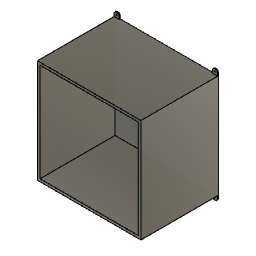
caixinha morea v0 (Autodesk Fusion 360 design; units mm, degrees)
Autodesk Fusion 360 part; units mm, degrees
note: some values were not read from the file. Chosen so that the rebuilt part matches the saved one: which face or edge a step refers to; that a step has no effect; how an offset face is resized.
box "BoxPrimitive1" add length 200 width 200 height 150 placed x (0, 0, 1) y (1, 0, 0) z (0, 1, 0) at (0, 0, 0) makes body 1
shell "Shell1" thickness 5 removed faces 1 at (133.3333, 0, 66.6667) on bodies 1
fillet "Fillet1" [no effect]
fillet "Fillet2" [no effect]
cylinder "CylinderPrimitive1" add diameter 40 height 200 placed x (1, 0, 0) y (0, 0, -1) z (0, 1, 0) at (-160, 0, 30) separate body makes body 2
delete_face "DeleteFace1" 3 faces at (-155.2577, 200, 37.1112) (-140.0994, 133.3333, 31.9914) (-155.2577, 0, 37.1112) on bodies 2
hole "Hole1" at (97.506, 145, 43.5548) direction (0, 1, 0) diameter 17 depth 80 tip angle 118 bodies 1
sketch "Sketch3" plane through (0, 150, 0) normal (0, 1, 0) x (-1, 0, 0)
  circle A0 centre (-97.506, 43.5548) radius 8.5
  line L0 (-200, 0) -> (0, 0)
  line L1 (0, 0) -> (0, 200)
  line L2 (0, 200) -> (-200, 200)
  line L3 (-200, 200) -> (-200, 0)
torus "TorusPrimitive1" cut centre line diameter 20 section diameter 13 placed x (1, 0, 0) y (0, 0, -1) z (0, 1, 0) at (200, 0, 175) bodies 1
delete_face "DeleteFace2" 1 faces at (196.1038, 1.3394, 190.8898) on bodies 1
hole "Hole3" at (188.159, 0, 189.1481) direction (0, 1, 0) diameter 7 depth 30 tip angle 118 bodies 1
thread "Thread3" "ISO Metric profile 7.0 M7x1 6H"
hole "Hole4" at (185.3643, 0, 8.9695) direction (0, 1, 0) diameter 7 depth 30 tip angle 118 bodies 1
thread "Thread4" "ISO Metric profile 7.0 M7x1 6H"
moveface "MoveFace1" [no effect]
moveface "MoveFace2" [no effect]
moveface "MoveFace3" [no effect]
moveface "MoveFace4" [no effect]
hole "Hole5" at (11.9529, 0, 10.7696) direction (0, 1, 0) diameter 7 depth 30 tip angle 118 bodies 1
thread "Thread5" "ISO Metric profile 7.0 M7x1 6H"
hole "Hole6" at (11.2095, 0, 187.8943) direction (0, 1, 0) diameter 7 depth 30 tip angle 118 bodies 1
thread "Thread6" "ISO Metric profile 7.0 M7x1 6H"
box "Primitiva de caixa3" add length 5 width 10 height 10 placed x (0, -1, 0) y (1, 0, 0) z (0, 0, 1) at (170, 100, 200) bodies 1
delete_face "Excluir face3" 5 faces at (173.3333, 100, 203.3333) (170, 96.6667, 203.3333) (173.3333, 95, 203.3333) (180, 96.6667, 203.3333) (176.6667, 98.3333, 210) on bodies 1
box "Primitiva de caixa4" add length 10 width 10 height 2 placed x (0, 0, -1) y (-1, 0, 0) z (0, 1, 0) at (150, 150, 220) separate body makes body 3
move_body "Mover9" bodies 3 to x (1, 0, 0) y (0, 1, 0) z (0, 0, 1) at (50, -2, -10)
hole "Furo7" at (195, 148, 205) direction (0, 1, 0) diameter 3 depth 5 tip angle 118 bodies 3
thread "Rosca7" "ISO Metric profile 2.0 M2x0.4 6H" major diameter 2.074 minor diameter 1.623 pitch 0.4 angle 60 resizes the face on face at (193.74, 148.6667, 204.1862) on bodies 3
fillet "Arredondamento4" radius 5 1 edges at (190, 149, 210) on bodies 3
fillet "Arredondamento5" radius 5 1 edges at (200, 149, 210) on bodies 3
copy_body "Copiar e colar corpos4" bodies 3 makes body 4
move_body "Mover10" bodies 4 to x (1, 0, 0) y (0, 1, 0) z (0, 0, 1) at (-190, 0, 0)
copy_body "Copiar e colar corpos5" bodies 4 makes body 5
move_body "Mover11" bodies 5 to x (0.996195, 0.087156, 0) y (0.087156, -0.996195, 0) z (0, 0, -1) at (-12.899, 295.4368, 400)
move_body "Mover12" bodies 5 to x (1, 0, 0) y (0, 1, 0) z (0, 0, 1) at (0, 0.9266, -199.427)
move_body "Mover13" bodies 5 to x (1, 0, 0) y (0, 1, 0) z (0, 0, 1) at (0, 0.2137, -0.5522)
move_body "Mover14" bodies 5 to x (0.996195, -0.087156, 0) y (0.087156, 0.996195, 0) z (0, 0, 1) at (-12.7376, 1.5561, 0)
move_body "Mover15" bodies 5 to x (1, 0, 0) y (0, 1, 0) z (0, 0, 1) at (-0.2018, -0.1367, -0.0651)
copy_body "Copiar e colar corpos6" bodies 5 makes body 6
move_body "Mover16" bodies 6 to x (1, 0, 0) y (0, 1, 0) z (0, 0, 1) at (190, 0, 0)
named bodies: "caixinha principal"
